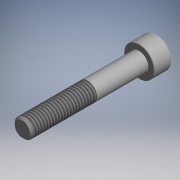
# Autodesk Inventor part: DIN-912 - M8x50(F)
Saved by Autodesk Inventor 2017.3 (Build 213256000, 256)
## iProperties
Part Number: DIN-912 - M8x50(F)
Material: Generic
Catalog Web Link: www.cadenas.de
Description: DIN-912-Cylinder screw
Vendor: FESTO
Document SubType Name: Modeling
Designer: partserver
Manufacturer: FESTO
Mass: 3.41329 g
Surface Area: 18.9476 cm^2
Volume: 3.41329 cm^3
Density: 1 g/cm^3
Appearance: PSOLRGB-192-192-192
Category: PARTsolutions
Company: FESTO
Title: DIN-912 - M8x50(F)
Author: Cadenas PARTsolutions
Comments: Cylinder screw
PSOL_IDENT_0: {$CADENAS_DATA\23d-libs\festo\zyl_zubeh\d912\din_912.prj},178 {VTYP=3D},{NB=DIN-912 - M8x50(F)},{LIN
PSOL_IDENT_1: A=DIN-912 - M8x50(F)},{NN=DIN-912},{DATE=01.07.2020 05:33:41},{GEOMDATE=01.07.2020 05:33:34},{VERSIO
PSOL_IDENT_2: N=},{LINEID=650},{WBVAR=},{WBNUMERIC=}  {NB=DIN-912 - M8x50(F)},{LINA=DIN-912 - M8x50(F)},{KT=X},{ID
PSOL_IDENT_3: NR=},{GEW=M8},{DG=8.000},{P=1.250},{L=50.000},{B=28.000},{FORM=0},{GKD=6.466},{DK=13.000},{DADIN=9.2
PSOL_IDENT_4: 00},{DS=8.000},{E=6.860},{LF=1.020},{K=8.000},{R=0.400},{S=6.000},{T=4.000},{V=0.800},{DW=12.330},{W=
PSOL_IDENT_5: 3.000},{NENN=M8x50},{DA=8.1},{BL=28}
NB: DIN-912 - M8x50(F)
NN: DIN-912
NT: Cylinder screw
NBSYN: DIN-912 - $NENN.(F)
LINA: DIN-912 - M8x50(F)
CATALOG: Festo
ROWDESC: M8x50
GEW: M8
DG: 8
P: 1.25
L: 50
B: 28
FORM: 0
GKD: 6.466
DK: 13
DADIN: 9.2
DS: 8
E: 6.86
LF: 1.02
K: 8
R: 0.4
S: 6
T: 4
V: 0.8
DW: 12.33
W: 3
SUPPLIER: FESTO
ARTICLENO: DIN-912 - M8x50(F)
BOMINFO: DIN-912 - M8x50(F)
CREATOR: CADENAS GmbH
Autodesk Inventor part; units mm, degrees
sketch "Sketch_1" plane through (0, 0, 0) normal (0, 0, 1) x (1, 0, 0)
  line L0 (0, -50) -> (0, 8)
  line L1 (0, 2.2679) -> (3, 4)
  line L2 (3, 4) -> (3, 7.5359)
  line L3 (3, 7.5359) -> (3.4641, 8)
  line L4 (3.4641, 8) -> (5.7, 8)
  line L5 (5.7, 8) -> (6.5, 7.2)
  line L6 (6.5, 7.2) -> (6.5, 0.2)
  line L7 (6.5, 0.2) -> (6.3, 0)
  line L8 (6.3, 0) -> (4.05, 0)
  line L9 (4.05, 0) -> (4, -1.02)
  line L10 (4, -1.02) -> (4, -49.233)
  line L11 (4, -49.233) -> (3.233, -50)
  line L12 (3.233, -50) -> (0, -50)
  line L13 (0, -50) -> (0, 2.2679)
  constraints: 28 end point
revolve "Revolution1" add sketch "Sketch_1" angle 360 about axis through (0, -50, 0) along (0, -1, 0)
thread "Thread1" size "M8x1.25" class "6g" standard "ISO Metric profile" length 27.233
sketch "Sketch_2" plane through (0, 8, 0) normal (0, 1, 0) x (1, 0, 0)
  line L0 (-3, -1.7321) -> (0, -3.4641)
  line L1 (0, -3.4641) -> (3, -1.7321)
  line L2 (3, -1.7321) -> (3, 1.7321)
  line L3 (3, 1.7321) -> (0, 3.4641)
  line L4 (0, 3.4641) -> (-3, 1.7321)
  line L5 (-3, 1.7321) -> (-3, -1.7321)
  constraints: 12 end point
extrude "Extrusion1" cut sketch "Sketch_2" against normal blind 4
ref_plane "ANBAU_XY" through (0, 0, 0) normal (0, 1, 0) x (1, 0, 0)
ref_plane "ANBAU_YZ" through (0, 0, 0) normal (1, 0, 0) x (0, 0, -1)
ref_plane "ANBAU_ZX" through (0, 0, 0) normal (0, 0, -1) x (0, 1, 0)
ref_plane "Schraube_XY" through (0, 0, 0) normal (0, 1, 0) x (1, 0, 0)
ref_plane "Schraube_YZ" through (0, 0, 0) normal (1, 0, 0) x (0, 0, -1)
ref_plane "Schraube_ZX" through (0, 0, 0) normal (0, 0, -1) x (0, 1, 0)
ref_plane "insert_XY" through (0, 0, 0) normal (0, 1, 0) x (1, 0, 0)
ref_plane "insert_YZ" through (0, 0, 0) normal (1, 0, 0) x (0, 0, -1)
ref_plane "insert_ZX" through (0, 0, 0) normal (0, 0, -1) x (0, 1, 0)
ref_plane "schrauben_punkt_XY" through (0, -50, 0) normal (0, 1, 0) x (1, 0, 0)
ref_plane "schrauben_punkt_YZ" through (0, -50, 0) normal (1, 0, 0) x (0, 0, -1)
ref_plane "schrauben_punkt_ZX" through (0, -50, 0) normal (0, 0, -1) x (0, 1, 0)
body "Solid1"
